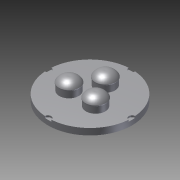
# Autodesk Inventor part: Top4
Saved by Autodesk Inventor 2012 (Build 160160000, 160)
## iProperties
Created: 2015-08-07
Part Number: Top4
Material: Default
Document SubType Name: Modeling
Designer: Craig
Density: 1 g/cm^3
Autodesk Inventor part; units mm, degrees
ref_plane "YZ Plane" through (0, 0, 0) normal (1, 0, 0) x (0, 1, 0)
ref_plane "XZ Plane" through (0, 0, 0) normal (0, 1, 0) x (-1, 0, 0)
ref_plane "XY Plane" through (0, 0, 0) normal (0, 0, 1) x (1, 0, 0)
sketch "Sketch3" plane through (0, 0, 0) normal (0, 0, 1) x (1, 0, 0)
  circle A0 centre (0, 0) radius 13
  dimension "d0" = 26
  constraints: 1 centre point, 1 coincident
  measures "d0" diameter of A0
extrude "Extrusion1" add sketch "Sketch3" along normal blind 2
sketch "Sketch4" plane through (0, 0, 2) normal (0, 0, 1) x (1, 0, 0)
  circle A0 centre (0, 0) radius 13 projected
  circle A1 centre (0, 4.75) radius 3
  line L0 (1.4999, 2.1519) -> (2.6135, 0.2228)
  line L1 (1.1135, -2.3753) -> (-1.1135, -2.3753)
  circle A2 centre (-4.1135, -2.3753) radius 3
  circle A3 centre (4.1135, -2.3753) radius 3
  arc A4 (-2.8465, 3.8026) -> (-4.7165, 0.5635) centre (0, 0) ccw
  arc A5 (-1.8696, -4.3666) -> (1.8696, -4.3666) centre (0, 0) ccw
  arc A6 (4.7165, 0.5635) -> (2.8465, 3.8026) centre (0, 0) ccw
  dimension "d4" = 6
  dimension "d5" = 6
  dimension "d6" = 6
  constraints: 16 point on circle, 6 centre point, 4 end point, 1 coincident, 1 horizontal
  measures "d4" diameter of A1
  measures "d5" diameter of A2
  measures "d6" diameter of A3
extrude "Extrusion2" add sketch "Sketch4" along normal blind 2 contours A1 | A2 | A3
sketch "Sketch5" plane through (-4.1135, -2.3753, 4) normal (0, 0, 1) x (1, 0, 0)
  circle A0 centre (0, 0) radius 3 projected
  circle A1 centre (4.1135, 7.1253) radius 3 projected
  circle A2 centre (8.2269, 0) radius 3 projected
  circle A3 centre (0, 0) radius 3.3
  circle A4 centre (4.1135, 7.1253) radius 3.3
  circle A5 centre (8.2269, 0) radius 3.3
  point P0 (4.1135, 2.3753)
  dimension "d9" = 6.6
  dimension "d10" = 6.6
  dimension "d11" = 6.6
  constraints: 3 centre point, 3 coincident
  measures "d9" diameter of A3
  measures "d10" diameter of A4
  measures "d11" diameter of A5
extrude "Extrusion3" add sketch "Sketch5" along normal blind 2 contours A0 | A1 | A2 | A3 | A4 | A5
fillet "Fillet1" radius 3.175 3 edges at (-7.4135, -2.3753, 6) (-3.3, 4.75, 6) (0.8135, -2.3753, 6)
fillet "Fillet2" radius 0.25 3 edges at (-7.4135, -2.3753, 4) (0.8135, -2.3753, 4) (-3.3, 4.75, 4)
sketch "Sketch9" plane through (0, 0, 0) normal (0, 0, -1) x (-1, 0, 0)
  circle A0 centre (0, 0) radius 13 projected
  circle A1 centre (0, 0) radius 0.9
  dimension "d25" = 1.8
  constraints: 1 centre point, 1 coincident
  measures "d25" diameter of A1
extrude "Extrusion7" cut sketch "Sketch9" against normal through all contours A1
sketch "Sketch11" plane through (0, 0, 2) normal (0, 0, 1) x (1, 0, 0)
  circle A0 centre (0, 0) radius 13 projected
  circle A1 centre (0, 13) radius 1
  circle A2 centre (13, 0) radius 1
  circle A3 centre (0, -13) radius 1
  circle A4 centre (-13, 0) radius 1
  dimension "d32" = 2
  dimension "d33" = 2
  dimension "d34" = 2
  dimension "d35" = 2
  constraints: 4 centre point, 4 point on circle
  measures "d32" diameter of A1
  measures "d33" diameter of A2
  measures "d34" diameter of A3
  measures "d35" diameter of A4
extrude "Extrusion8" cut sketch "Sketch11" against normal blind 0.5 contours A0 A2 | A0 A2 | A1 A0 | A0 A1 | A3 A0 | A0 A3 | A4 A0 | A0 A4
body "Solid1"
